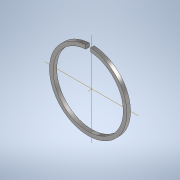
# Autodesk Inventor part: piston ring
Saved by Autodesk Inventor 2021.1 (Build 251245000, 245)
## iProperties
Created: 2020-08-31
Part Number: piston ring
Material: Stainless Steel
Document SubType Name: Sheet Metal
Designer: Vamshi
Mass: 27.673 g
Surface Area: 36.6072 cm^2
Volume: 3.45912 cm^3
Density: 8 g/cm^3
Sheet Metal Rule: Default
Appearance: Semi-Polished
Author: Vamshi
Autodesk Inventor part; units mm, degrees
ref_plane "YZ Plane" through (0, 0, 0) normal (1, 0, 0) x (0, 1, 0)
ref_plane "XZ Plane" through (0, 0, 0) normal (0, 1, 0) x (-1, 0, 0)
ref_plane "XY Plane" through (0, 0, 0) normal (0, 0, 1) x (1, 0, 0)
sketch "Sketch1" plane through (0, 0, 0) normal (0, 0, 1) x (1, 0, 0)
  arc A0 (-2.54, 36.7423) -> (2.54, 36.7423) centre (0, 0) ccw
  arc A1 (-2.54, 40.5605) -> (2.54, 40.5605) centre (0, 0) ccw
  line L0 (-2.54, 40.5605) -> (-2.54, 36.7423)
  line L1 (2.54, 40.5605) -> (2.54, 36.7423)
  line L2 (0, -56.8801) -> (0, 56.8007) projected
  dimension "d0" = 73.66
  dimension "d1" = 81.28
  dimension "d2" = 5.08
  constraints: 4 end point, 4 point on circle, 2 centre point, 2 coincident, 2 vertical, 1 other
  measures "d0" diameter of A0
  measures "d1" diameter of A1
  measures "d2" distance between parallel lines of L1 L0
extrude "Extrusion1" add sketch "Sketch1" along normal blind 3.81
equation "\"BendRadius\" = Thickness"
equation "\"BendReliefWidth\" = Thickness"
equation "\"BendReliefDepth\" = 0.5 * Thickness"
equation "\"CornerReliefSize\" = 4 * Thickness"
equation "\"MinimumRemnant\" = 2 * Thickness"
equation "\"TransitionRadius\" = BendRadius"
equation "\"JacobiRadiusSize\" = BendRadius"
equation "\"GapSize\" = Thickness"
equation "\"Thickness\" = 3.048"
body "Solid1"
